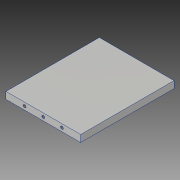
# Autodesk Inventor part: motor_base_plate
Saved by Autodesk Inventor 2019 (Build 230136000, 136)
## iProperties
Created: 2018-09-24
Part Number: motor_base_plate
Material: Aluminum 6061
Document SubType Name: Modeling
Designer: Callum Snowden
Mass: 390.482 g
Surface Area: 351.399 cm^2
Volume: 144.623 cm^3
Density: 2.7 g/cm^3
Appearance: Aluminum - Flat
Author: Callum Snowden
Autodesk Inventor part; units mm, degrees
ref_plane "YZ Plane" through (0, 0, 0) normal (1, 0, 0) x (0, 1, 0)
ref_plane "XZ Plane" through (0, 0, 0) normal (0, 1, 0) x (-1, 0, 0)
ref_plane "XY Plane" through (0, 0, 0) normal (0, 0, 1) x (1, 0, 0)
sketch "Sketch1" plane through (0, 0, 0) normal (0, 1, 0) x (-1, 0, 0)
  line L0 (54, -67.5) -> (-54, -67.5)
  line L1 (-54, -67.5) -> (-54, 67.5)
  line L2 (-54, 67.5) -> (54, 67.5)
  line L3 (54, 67.5) -> (54, -67.5)
  line L4 (0, -94.5) -> (0, 94.5) construction
  line L5 (-75.6, 0) -> (75.6, 0) construction
  point P0 (0, 0)
  dimension "d0" = 108
  dimension "d1" = 135
  constraints: 8 end point, 2 parallel, 1 horizontal, 1 perpendicular, 2 other
  measures "d0" distance of L1.end L2.end
  measures "d1" distance of L0.end L1.end
extrude "Extrusion1" add sketch "Sketch1" along normal blind 10
sketch "Sketch2" plane through (-54, 0, 67.5) normal (0, 0, 1) x (1, 0, 0)
  line L0 (108, 10) -> (0, 10) projected
  line L1 (54, 10) -> (54, 0) construction
  line L2 (3.9342, 5) -> (111.9342, 5) construction
  point P0 (54, 5)
  point P1 (81, 5)
  point P2 (27, 5)
  dimension "d4" = 54
  constraints: 4 end point, 2 midpoint, 2 point on line, 1 horizontal, 1 symmetric about line, 1 vertical
  measures "d4" distance of point (81, 5) point (27, 5)
hole "Hole1" at (0, 5, 67.5) at (27, 5, 67.5) at (-27, 5, 67.5) direction (0, 0, -1) diameter 4.134 depth 14.2 tip angle 118 thread size "M5x0.8" class "6H" standard "ISO Metric profile"
sketch "Sketch3" plane through (54, 0, -67.5) normal (0, 0, -1) x (-1, 0, 0)
  point P0 (54, 0)
  point P1 (27, 5)
  point P2 (54, 5)
  point P3 (81, 5)
hole "Hole2" at (27, 5, -67.5) at (0, 5, -67.5) at (-27, 5, -67.5) direction (0, 0, 1) diameter 4.134 depth 14.2 tip angle 118 thread size "M5x0.8" class "6H" standard "ISO Metric profile"
body "Solid1"
